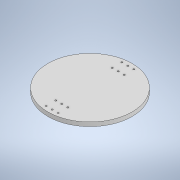
# Autodesk Inventor part: Base do tripé
Saved by Autodesk Inventor 2021 (Build 250183000, 183)
## iProperties
Created: 2021-08-09
Part Number: Base do tripé
Material: Generic
Document SubType Name: Modeling
Designer: guilh
Density: 1 g/cm^3
Appearance: Default
Author: guilh
Autodesk Inventor part; units mm, degrees
ref_plane "YZ Plane" through (0, 0, 0) normal (1, 0, 0) x (0, 1, 0)
ref_plane "XZ Plane" through (0, 0, 0) normal (0, 1, 0) x (-1, 0, 0)
ref_plane "XY Plane" through (0, 0, 0) normal (0, 0, 1) x (1, 0, 0)
sketch "Sketch1" plane through (0, 0, 0) normal (0, 1, 0) x (-1, 0, 0)
  circle A0 centre (0, 0) radius 105
  dimension "d0" = 210
  constraints: 1 centre point, 1 coincident
  measures "d0" diameter of A0
extrude "Extrusion1" add sketch "Sketch1" along normal blind 10
sketch "Sketch2" plane through (0, 10, 0) normal (0, 1, 0) x (1, 0, 0)
  circle A0 centre (0, 0) radius 2.5
  dimension "d3" = 5
  constraints: 1 centre point, 1 coincident
  measures "d3" diameter of A0
extrude "Extrusion2" cut sketch "Sketch2" against normal blind 10
sketch "Sketch3" plane through (0, 10, 0) normal (0, 1, 0) x (1, 0, 0)
  circle A0 centre (0, 0) radius 2.5 projected
  line L0 (0, 0) -> (0, -75)
  line L1 (0, -75) -> (-15, -75)
  circle A1 centre (-30, 0) radius 2.5
  circle A2 centre (-15, 0) radius 2.5
  circle A3 centre (0, 0) radius 2.5
  line L2 (15, 70.5) -> (15, 94.5)
  line L3 (0, 0) -> (29.6742, 0)
  line L4 (15, -70.5) -> (15, -94.5)
  circle A4 centre (-15, 70.5) radius 2.5
  circle A5 centre (0, 70.5) radius 2.5
  circle A6 centre (15, 70.5) radius 2.5
  circle A7 centre (-15, 94.5) radius 2.5
  circle A8 centre (0, 94.5) radius 2.5
  circle A9 centre (15, 94.5) radius 2.5
  circle A10 centre (-15, -70.5) radius 2.5
  circle A11 centre (0, -70.5) radius 2.5
  circle A12 centre (15, -70.5) radius 2.5
  circle A13 centre (-15, -94.5) radius 2.5
  circle A14 centre (0, -94.5) radius 2.5
  circle A15 centre (15, -94.5) radius 2.5
  dimension "d9" = 75
  dimension "d10" = 15
  dimension "d19" = 5
  dimension "d20" = 5
  dimension "d21" = 5
  dimension "d25" = 5
  dimension "d26" = 5
  dimension "d27" = 5
  dimension "d28" = 5
  dimension "d29" = 5
  dimension "d30" = 5
  dimension "d31" = 5
  dimension "d32" = 5
  dimension "d33" = 5
  dimension "d34" = 5
  dimension "d35" = 5
  dimension "d36" = 5
  constraints: 15 centre point, 10 end point, 2 symmetric about line, 2 vertical, 1 horizontal, 1 perpendicular
  measures "d9" distance of L0.start L0.end
  measures "d10" distance of L0.end L1.end
  measures "d19" diameter of A1
  measures "d20" diameter of A2
  measures "d21" diameter of A3
  measures "d25" diameter of A4
  measures "d26" diameter of A5
  measures "d27" diameter of A6
  measures "d28" diameter of A7
  measures "d29" diameter of A8
  measures "d30" diameter of A9
  measures "d31" diameter of A10
  measures "d32" diameter of A11
  measures "d33" diameter of A12
  measures "d34" diameter of A13
  measures "d35" diameter of A14
  measures "d36" diameter of A15
extrude "Extrusion3" cut sketch "Sketch3" against normal blind 10 contours A11 L0 | L0 A11 | A9 | A6 | A15 | A12 | A4 | A5 | A7 | A8 | A10 | A13 | A14
sketch "Sketch4" plane through (0, 10, 0) normal (0, 1, 0) x (1, 0, 0)
  circle A0 centre (-15, 94.5) radius 2
  circle A1 centre (0, 94.5) radius 2
  circle A2 centre (15, 94.5) radius 2
  circle A3 centre (15, 70.5) radius 2
  circle A4 centre (0, 70.5) radius 2
  circle A5 centre (-15, 70.5) radius 2
  circle A6 centre (15, -70.5) radius 2
  circle A7 centre (15, -94.5) radius 2
  circle A8 centre (0, -94.5) radius 2
  circle A9 centre (-15, -94.5) radius 2
  circle A10 centre (-15, -70.5) radius 2
  circle A11 centre (0, -70.5) radius 2
  line L0 (-22.4241, -99.4431) -> (24.1315, -99.4431)
  line L1 (24.1315, -99.4431) -> (24.1315, 99.2987)
  line L2 (24.1315, 99.2987) -> (-24.4086, 99.2987)
  line L3 (-24.4086, 99.2987) -> (-22.4241, -99.4431)
  point P0 (0, 0)
  dimension "d39" = 4
  dimension "d40" = 4
  dimension "d41" = 4
  dimension "d42" = 4
  dimension "d43" = 4
  dimension "d44" = 4
  dimension "d45" = 4
  dimension "d46" = 4
  dimension "d47" = 4
  dimension "d48" = 4
  dimension "d49" = 4
  dimension "d50" = 4
  constraints: 12 centre point, 9 coincident, 8 end point, 2 perpendicular, 1 horizontal
  measures "d39" diameter of A0
  measures "d40" diameter of A1
  measures "d41" diameter of A2
  measures "d42" diameter of A3
  measures "d43" diameter of A4
  measures "d44" diameter of A5
  measures "d45" diameter of A6
  measures "d46" diameter of A7
  measures "d47" diameter of A8
  measures "d48" diameter of A9
  measures "d49" diameter of A10
  measures "d50" diameter of A11
extrude "Extrusion4" add sketch "Sketch4" against normal blind 10
body "Solid1"
